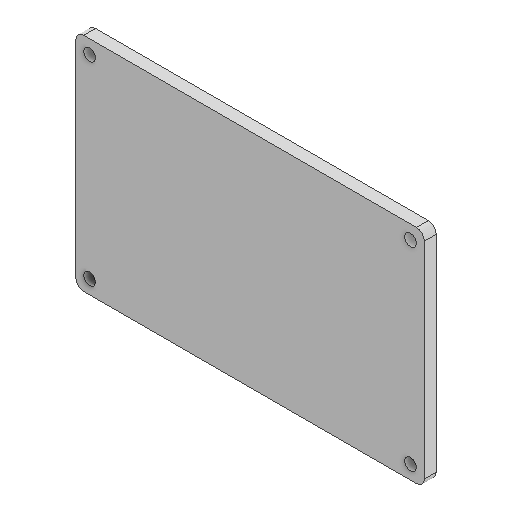
# Autodesk Inventor part: Distance_plate
Saved by Autodesk Inventor 2025.2 (Build 292293000, 293)
## iProperties
Created: 2025-03-12
Part Number: Distance_plate
Material: Generic
Document SubType Name: Modeling
Designer: ahorat
Density: 1 g/cm^3
Appearance: Default
Author: ahorat
Autodesk Inventor part; units mm, degrees
ref_plane "YZ Plane" through (0, 0, 0) normal (1, 0, 0) x (0, 1, 0)
ref_plane "XZ Plane" through (0, 0, 0) normal (0, 1, 0) x (-1, 0, 0)
ref_plane "XY Plane" through (0, 0, 0) normal (0, 0, 1) x (1, 0, 0)
sketch "Sketch1" plane through (0, 0, 0) normal (0, 0, 1) x (1, 0, 0)
  line L0 (-44, -28) -> (44, -28)
  line L1 (44, -28) -> (44, 28)
  line L2 (44, 28) -> (-44, 28)
  line L3 (-44, 28) -> (-44, -28)
  line L4 (-44, -28) -> (44, 28) construction
  line L5 (44, -28) -> (-44, 28) construction
  point P0 (0, 0)
  dimension "d0" = 88
  dimension "d1" = 56
  constraints: 12 end point, 2 midpoint, 2 parallel, 1 horizontal, 1 perpendicular
  measures "d0" distance of L1.end L2.end
  measures "d1" distance of L0.end L1.end
extrude "Extrusion1" add sketch "Sketch1" along normal blind 3
fillet "Fillet1" radius 2 4 edges at (44, 28, 1.5) (44, -28, 1.5) (-44, 28, 1.5) (-44, -28, 1.5)
sketch "Sketch2" plane through (0, 0, 3) normal (0, 0, 1) x (1, 0, 0)
  line L0 (-40.5, -24.5) -> (40.5, -24.5)
  line L1 (40.5, -24.5) -> (40.5, 24.5)
  line L2 (40.5, 24.5) -> (-40.5, 24.5)
  line L3 (-40.5, 24.5) -> (-40.5, -24.5)
  line L4 (-40.5, -24.5) -> (40.5, 24.5) construction
  line L5 (40.5, -24.5) -> (-40.5, 24.5) construction
  point P0 (0, 0)
  point P1 (-40.5, 24.5)
  dimension "d12" = 81
  dimension "d13" = 49
  constraints: 12 end point, 4 coincident, 2 midpoint, 2 parallel, 1 horizontal, 1 perpendicular
  measures "d12" distance of L1.end L2.end
  measures "d13" distance of L0.end L1.end
hole "Hole1" at (-40.5, -24.5, 3) at (-40.5, 24.5, 3) at (40.5, -24.5, 3) at (40.5, 24.5, 3) direction (0, 0, -1) diameter 3 end through all
body "Solid1"
